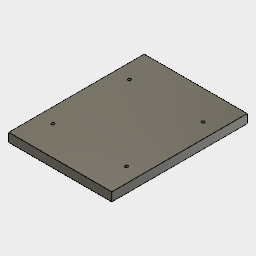
_motor_tip_hold_3D.4e5e734c-ea4f-4d34-8a0c-042d3958b99a (Autodesk Fusion 360 design; units mm, degrees)
Autodesk Fusion 360 part; units mm, degrees
sketch "Sketch1" plane through (0, 0, 0) normal (0, 1, 0) x (1, 0, 0)
  line L0 (17.5, 23) -> (-17.5, 23)
  line L1 (-17.5, 23) -> (-17.5, -23)
  line L2 (-17.5, -23) -> (17.5, -23)
  line L3 (17.5, -23) -> (17.5, 23)
  line L4 (17.5, 23) -> (-17.5, -23) construction
  line L5 (-17.5, 23) -> (17.5, -23) construction
  circle A0 centre (-12.5, -13) radius 0.5
  circle A1 centre (12.5, -13) radius 0.5
  circle A2 centre (12.5, 13) radius 0.5
  circle A3 centre (-12.5, 13) radius 0.5
  dimension "d1" = 46
  dimension "d2" = 35
  dimension "d3" = 1
  dimension "d4" = 1
  dimension "d5" = 1
  dimension "d6" = 1
  dimension "d7" = 10
  dimension "d8" = 5
  dimension "d9" = 5
  dimension "d10" = 10
  dimension "d11" = 10
  dimension "d12" = 5
  dimension "d13" = 10
  dimension "d14" = 5
  dimension "d15" = 15
  dimension "d16" = 15
  measures "d1" distance of L0.end L1.end
  measures "d2" distance of L1.end L2.end
  measures "d3" diameter of A0
  measures "d4" diameter of A1
  measures "d5" diameter of A2
  measures "d6" diameter of A3
  measures "d7" distance of L0 A3.centre
  measures "d8" distance of L1 A3.centre
  measures "d9" distance of L3 A2.centre
  measures "d10" distance of L0 A2.centre
  measures "d11" distance of L2 A1.centre
  measures "d12" distance of L3 A1.centre
  measures "d13" distance of L2 A0.centre
  measures "d14" distance of L1 A0.centre
extrude "Extrude1" add sketch "Sketch1" along normal blind 3
